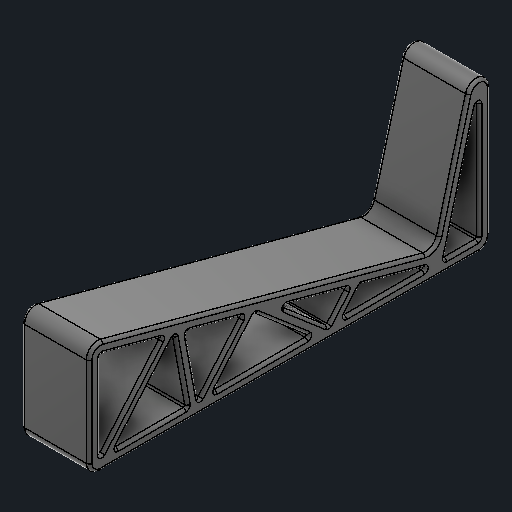
# Autodesk Inventor part: Amp Stand
Saved by Autodesk Inventor 2026.2 (Build 302298000, 298)
## iProperties
Created: 2026-07-31
Part Number: Amp Stand
Material: ABS Plastic
Document SubType Name: Modeling
Designer: JoshuaEah
Density: 1.06 g/cm^3
Appearance: Smooth - Black
Author: JoshuaEah
Autodesk Inventor part; units mm, degrees
ref_plane "YZ Plane" through (0, 0, 0) normal (1, 0, 0) x (0, 1, 0)
ref_plane "XZ Plane" through (0, 0, 0) normal (0, 1, 0) x (-1, 0, 0)
ref_plane "XY Plane" through (0, 0, 0) normal (0, 0, 1) x (1, 0, 0)
sketch "Sketch1" plane through (0, 0, 0) normal (1, 0, 0) x (0, 1, 0)
  line L0 (0, 0) -> (0, -226.8383)
  line L1 (0, 0) -> (65.292, 0)
  line L2 (65.292, 0) -> (12.7, -196.2761)
  line L3 (12.7, -196.2761) -> (86.3035, -215.9981)
  line L4 (86.3035, -215.9981) -> (83.3989, -226.8383)
  line L5 (83.3989, -226.8383) -> (0, -226.8383)
  line L6 (78.5264, -220.4883) -> (6.35, -201.1487)
  line L7 (6.35, -201.1487) -> (6.35, -220.4883)
  line L8 (6.35, -220.4883) -> (78.5264, -220.4883)
  line L9 (57.0165, -6.35) -> (6.35, -6.35)
  line L10 (6.35, -6.35) -> (47.5602, -41.6416)
  line L11 (47.5602, -41.6416) -> (57.0165, -6.35)
  line L12 (45.7381, -48.4416) -> (6.35, -14.7103)
  line L13 (6.35, -14.7103) -> (6.35, -55.7959)
  line L14 (6.35, -55.7959) -> (45.7381, -48.4416)
  line L15 (43.9161, -55.2415) -> (6.35, -62.2556)
  line L16 (43.9161, -55.2415) -> (35.3761, -87.1131)
  line L17 (35.3761, -87.1131) -> (6.35, -62.2556)
  line L18 (33.5541, -93.913) -> (6.35, -70.6159)
  line L19 (6.35, -70.6159) -> (6.35, -125.6794)
  line L20 (6.35, -125.6794) -> (33.5541, -93.913)
  line L21 (29.7471, -108.1208) -> (6.35, -135.4417)
  line L22 (6.35, -135.4417) -> (19.426, -146.6398)
  line L23 (19.426, -146.6398) -> (29.7471, -108.1208)
  line L24 (17.604, -153.4397) -> (6.35, -143.802)
  line L25 (6.35, -143.802) -> (6.35, -195.4401)
  line L26 (6.35, -195.4401) -> (17.604, -153.4397)
  point P0 (6.35, -195.4401)
  dimension "d1" = 203.2
  dimension "d2" = 76.2
  dimension "d12" = 6.35
  dimension "d13" = 6.35
  dimension "d14" = 6.35
  dimension "d15" = 12.7
  dimension "d16" = 6.35
  dimension "d24" = 15
  dimension "d25" = 6.35
  dimension "d26" = 6.35
  dimension "d27" = 6.35
  dimension "d28" = 6.35
  dimension "d29" = 6.35
  dimension "d30" = 64.424
  dimension "d31" = 64.424
  dimension "d32" = 6.35
  dimension "d33" = 6.35
  dimension "d34" = 6.35
  constraints: 54 end point, 15 point on line, 12 parallel, 5 perpendicular, 3 horizontal, 2 vertical, 1 coincident, 1 collinear
  measures "d1" distance of L1.end L2.end
  measures "d2" distance of L2.end L3.end
  measures "d12" distance between parallel lines of L3 L6
  measures "d13" distance between parallel lines of L5 L8
  measures "d14" distance between parallel lines of L0 L7
  measures "d15" distance from line of L0 L2.end
  measures "d16" distance from line of L4 L6.start
  measures "d24" angle of L0 L2
  measures "d25" distance between parallel lines of L2 L11
  measures "d26" distance between parallel lines of L1 L9
  measures "d27" distance between parallel lines of L12 L10
  measures "d28" distance between parallel lines of L15 L14
  measures "d29" distance between parallel lines of L0 L13
  measures "d30" angle of L2 L12
  measures "d31" angle of L2 L14
  measures "d32" distance between parallel lines of L17 L18
  measures "d33" distance between parallel lines of L21 L20
  measures "d34" distance between parallel lines of L22 L24
extrude "Extrusion1" add sketch "Sketch1" along normal blind 38.1
fillet "Fillet1" radius 6.35 6 edges at (19.05, 12.7, -196.2761) (19.05, 65.292, 0) (19.05, 0, 0) (19.05, 0, -226.8383) (19.05, 83.3989, -226.8383) (19.05, 86.3035, -215.9981)
fillet "Fillet1" radius 0.7937 21 edges at (19.05, 6.35, -201.1487) (19.05, 6.35, -220.4883) (19.05, 78.5264, -220.4883) (19.05, 57.0165, -6.35) (19.05, 6.35, -6.35) (19.05, 47.5602, -41.6416) (19.05, 45.7381, -48.4416) (19.05, 6.35, -55.7959) (19.05, 6.35, -14.7103) (19.05, 43.9161, -55.2415) (19.05, 6.35, -62.2556) (19.05, 35.3761, -87.1131) (19.05, 33.5541, -93.913) (19.05, 6.35, -70.6159) (19.05, 6.35, -125.6794) (19.05, 6.35, -135.4417) (19.05, 19.426, -146.6398) (19.05, 29.7471, -108.1208) (19.05, 17.604, -153.4397) (19.05, 6.35, -143.802) (19.05, 6.35, -195.4401)
fillet "Fillet2" radius 1.5875 92 edges at (38.1, 73.2849, -219.7982) (38.1, 39.8208, -220.4883) (38.1, 6.5825, -220.2558) (38.1, 6.35, -210.9388) (38.1, 6.6605, -201.5533) (38.1, 40.0263, -210.1722) (0, 6.5825, -220.2558) (0, 6.35, -210.9388) (0, 6.6605, -201.5533) (0, 40.0263, -210.1722) (0, 73.2849, -219.7982) (0, 39.8208, -220.4883) (0, 62.0544, -2.4843) (0, 1.8598, -1.8598) (0, 1.8598, -224.9784) (0, 84.0257, -217.3132) (0, 82.3921, -225.5261) (0, 84.6601, -222.1318) (0, 25.3289, -58.712) (38.1, 62.0544, -2.4843) (38.1, 1.8598, -1.8598) (38.1, 1.8598, -224.9784) (38.1, 84.0257, -217.3132) (38.1, 82.3921, -225.5261) (38.1, 84.6601, -222.1318) (38.1, 25.3289, -58.712) (38.1, 6.6366, -55.4509) (38.1, 6.35, -35.6376) (38.1, 6.8119, -15.7139) (38.1, 26.0693, -31.5975) (38.1, 44.729, -48.1712) (38.1, 25.6987, -52.1832) (0, 44.729, -48.1712) (0, 25.6987, -52.1832) (0, 6.6366, -55.4509) (0, 6.35, -35.6376) (0, 6.8119, -15.7139) (0, 26.0693, -31.5975) (38.1, 47.3545, -40.9776) (38.1, 27.292, -24.2844) (38.1, 7.7525, -6.8685) (38.1, 32.2396, -6.35) (38.1, 56.6119, -6.6605) (38.1, 52.3175, -23.887) (0, 47.3545, -40.9776) (0, 27.292, -24.2844) (0, 7.7525, -6.8685) (0, 32.2396, -6.35) (0, 56.6119, -6.6605) (0, 52.3175, -23.887) (38.1, 6.8685, -124.2769) (38.1, 6.35, -97.9365) (38.1, 6.8119, -71.6196) (38.1, 20.3056, -82.5673) (38.1, 33.2263, -93.9384) (38.1, 20.3922, -109.2823) (0, 20.3922, -109.2823) (0, 6.8685, -124.2769) (0, 6.35, -97.9365) (0, 6.8119, -71.6196) (0, 20.3056, -82.5673) (0, 33.2263, -93.9384) (38.1, 35.1704, -86.449) (38.1, 21.0144, -74.814) (38.1, 39.6461, -71.1773) (0, 35.1704, -86.449) (0, 21.0144, -74.814) (0, 39.6461, -71.1773) (38.1, 19.2203, -145.9757) (38.1, 12.711, -140.8892) (38.1, 6.6778, -135.4164) (38.1, 17.1695, -122.8078) (38.1, 28.4455, -110.5907) (38.1, 24.2971, -128.4606) (0, 19.2203, -145.9757) (0, 12.711, -140.8892) (0, 6.6778, -135.4164) (0, 17.1695, -122.8078) (0, 28.4455, -110.5907) (0, 24.2971, -128.4606) (38.1, 7.0401, -190.1986) (38.1, 6.35, -167.4692) (38.1, 6.8119, -144.8056) (38.1, 12.442, -149.0191) (38.1, 17.4661, -153.4824) (38.1, 12.6924, -171.7699) (0, 7.0401, -190.1986) (0, 6.35, -167.4692) (0, 6.8119, -144.8056) (0, 12.442, -149.0191) (0, 17.4661, -153.4824) (0, 12.6924, -171.7699)
fillet_without_effect "Fillet3"
body "Solid1"
